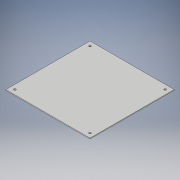
# Autodesk Inventor part: MAN_BASIS_PLATE
Saved by Autodesk Inventor 2019 (Build 230136000, 136)
## iProperties
Created: 2021-03-06
Part Number: MAN_BASIS_PLATE
Material: Generic
Document SubType Name: Modeling
Designer: DOMEK
Density: 1 g/cm^3
Appearance: Default
Author: DOMEK
Autodesk Inventor part; units mm, degrees
ref_plane "YZ Plane" through (0, 0, 0) normal (1, 0, 0) x (0, 1, 0)
ref_plane "XZ Plane" through (0, 0, 0) normal (0, 1, 0) x (-1, 0, 0)
ref_plane "XY Plane" through (0, 0, 0) normal (0, 0, 1) x (1, 0, 0)
sketch "Sketch1" plane through (0, 0, 0) normal (0, 1, 0) x (-1, 0, 0)
  line L0 (0, 0) -> (200, 0)
  line L1 (200, 0) -> (200, 200)
  line L2 (200, 200) -> (0, 200)
  line L3 (0, 200) -> (0, 0)
  dimension "d0" = 200
  dimension "d1" = 200
  constraints: 8 end point, 2 parallel, 1 horizontal, 1 perpendicular
  measures "d0" distance of L2.end L1.end
  measures "d1" distance of L1.end L0.end
extrude "Extrusion1" add sketch "Sketch1" along normal blind 2
sketch "Sketch2" plane through (0, 2, 0) normal (0, 1, 0) x (1, 0, 0)
  line L0 (-200, -200) -> (0, -200) projected
  line L1 (0, 0) -> (-200, 0) projected
  line L2 (0, -200) -> (0, 0) projected
  line L3 (-200, 0) -> (-200, -200) projected
  circle A0 centre (-10.6066, -189.3934) radius 2.5
  circle A1 centre (-189.3934, -189.3934) radius 2.5
  circle A2 centre (-10.6066, -10.6066) radius 2.5
  circle A3 centre (-189.3934, -10.6066) radius 2.5
  dimension "d9" = 5
  dimension "d10" = 5
  constraints: 4 centre point
  measures "d9" diameter of A1
  measures "d10" diameter of A2
extrude "Extrusion2" cut sketch "Sketch2" against normal blind 2 contours A0 | A1 | A2 | A3
body "Solid1"
